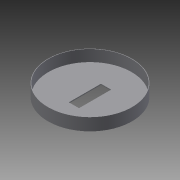
# Autodesk Inventor part: Bottom Cap
Saved by Autodesk Inventor 2015 (Build 190159000, 159)
## iProperties
Created: 2014-06-24
Part Number: Bottom Cap
Material: Generic
Document SubType Name: Modeling
Designer: Aki
Density: 1 g/cm^3
Appearance: Default
Author: Aki
Autodesk Inventor part; units mm, degrees
ref_plane "XZ Plane" through (0, 0, 0) normal (0, 1, 0) x (-1, 0, 0)
ref_plane "XY Plane" through (0, 0, 0) normal (0, 0, 1) x (1, 0, 0)
sketch "Sketch1" plane through (0, 0, 0) normal (0, 1, 0) x (-1, 0, 0)
  circle A0 centre (0, 0) radius 87
  line L0 (10.5, 33.25) -> (-10.5, 33.25)
  line L1 (-10.5, 33.25) -> (-10.5, -33.25)
  line L2 (-10.5, -33.25) -> (10.5, -33.25)
  line L3 (10.5, -33.25) -> (10.5, 33.25)
  line L4 (10.5, 33.25) -> (-10.5, -33.25) construction
  line L5 (-10.5, 33.25) -> (10.5, -33.25) construction
  dimension "d0" = 174
  dimension "d1" = 21
  dimension "d2" = 66.5
  constraints: 12 end point, 2 midpoint, 2 parallel, 1 centre point, 1 coincident, 1 horizontal, 1 perpendicular
  measures "d0" diameter of A0
  measures "d1" distance of L2.end L1.end
  measures "d2" distance of L1.end L0.end
ref_plane "Work Plane1" through (0, 0, 0) normal (1, 0, 0) x (0, 1, 0)
extrude "Extrusion2" add sketch "Sketch1" along normal blind 25.4
sketch "Sketch3" plane through (0, 25.4, 0) normal (0, 1, 0) x (1, 0, 0)
  circle A0 centre (0, 0) radius 86
  dimension "d63" = 172
  constraints: 1 centre point, 1 coincident
  measures "d63" diameter of A0
hole "Hole2" at (0, 25.4, 0) direction (0, -1, 0) diameter 172 depth 23.4
body "Solid2"
